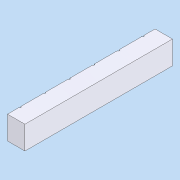
# Autodesk Inventor part: Nut
Saved by Autodesk Inventor 2021 (Build 250183000, 183)
## iProperties
Created: 2021-02-02
Part Number: Nut
Material: Generic
Document SubType Name: Modeling
Designer: garre
Density: 1 g/cm^3
Appearance: Default
Author: garre
Autodesk Inventor part; units mm, degrees
ref_plane "YZ Plane" through (0, 0, 0) normal (1, 0, 0) x (0, 1, 0)
ref_plane "XZ Plane" through (0, 0, 0) normal (0, 1, 0) x (-1, 0, 0)
ref_plane "XY Plane" through (0, 0, 0) normal (0, 0, 1) x (1, 0, 0)
sketch "Sketch1" plane through (0, 0, 0) normal (0, 1, 0) x (-1, 0, 0)
  line L0 (0, 0) -> (9, 0)
  line L1 (9, 0) -> (9, -76.2)
  line L2 (9, -76.2) -> (0, -76.2)
  line L3 (0, -76.2) -> (0, 0)
  dimension "d0" = 76.2
  dimension "d1" = 9
  constraints: 8 end point, 2 parallel, 1 horizontal, 1 perpendicular
  measures "d0" distance of L0.end L1.end
  measures "d1" distance of L1.end L2.end
extrude "Extrusion1" add sketch "Sketch1" against normal blind 6
extrude "Extrusion2" add sketch "Sketch1" along normal blind 6
sketch "Sketch2" plane through (0, 6, 0) normal (0, 1, 0) x (1, 0, 0)
  line L0 (-9, 0) -> (-9, 76.2) projected
  line L1 (0, 76.2) -> (0, 0) projected
  circle A0 centre (-9, 31.75) radius 0.5
  circle A1 centre (-9, 6.35) radius 0.5
  circle A2 centre (-9, 19.05) radius 0.5
  circle A3 centre (-9, 44.45) radius 0.5
  circle A4 centre (-9, 57.15) radius 0.5
  circle A5 centre (-9, 69.85) radius 0.5
  line L2 (-9, 76.2) -> (-9, 0) projected
  line L3 (-9, 0) -> (0, 0) projected
  dimension "d6" = 6.35
  dimension "d7" = 12.7
  dimension "d8" = 1
  dimension "d9" = 12.7
  dimension "d10" = 12.7
  dimension "d11" = 12.7
  dimension "d12" = 12.7
  constraints: 6 centre point, 5 equal radius, 5 point on line
  measures "d6" distance from line of L3 A1.centre
  measures "d7" distance of A2.centre A1.centre
  measures "d8" diameter of A1
  measures "d9" distance of A0.centre A2.centre
  measures "d10" distance of A3.centre A0.centre
  measures "d11" distance of A4.centre A3.centre
  measures "d12" distance of A5.centre A4.centre
extrude "Extrusion3" cut sketch "Sketch2" against normal up to surface (12 mm away)
equation "\"d0\" = nutLength"
equation "\"d1\" = nutWidth"
equation "\"d2\" = nutHeight"
equation "\"d4\" = nutHeight"
equation "\"d6\" = sideOffset"
equation "\"d7\" = holeOffset"
equation "\"d8\" = holeDiameter"
equation "\"d9\" = holeOffset"
equation "\"d10\" = holeOffset"
equation "\"d11\" = holeOffset"
equation "\"d12\" = holeOffset"
equation "\"d13\" = nutHeight"
equation "\"nutLength\" = 76.2"
equation "\"nutWidth\" = 9"
equation "\"nutHeight\" = 6"
equation "\"holeOffset\" = -0.4 * sideOffset + 0.2 * nutLength"
equation "\"sideOffset\" = 6.35"
equation "\"holeDiameter\" = 1"
body "Solid1"
